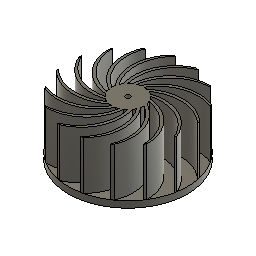
Hélice (Autodesk Fusion 360 design; units mm, degrees)
Autodesk Fusion 360 part; units mm, degrees
sketch "Sketch1" plane through (0, 0, 0) normal (0, 1, 0) x (1, 0, 0)
  circle A0 centre (0, 0) radius 5
  circle A1 centre (0, 0) radius 18.5
  circle A2 centre (0, 0) radius 0.75
  line L0 (-21, 0) -> (20.3872, 0) construction
  line L1 (0, 20) -> (0, -20) construction
  arc A3 (10.124, -15.484) -> (5, 0) centre (-1.6517, -10.791) ccw
  arc A4 (15.2788, -10.4311) -> (4.6194, 1.9134) centre (2.6036, -10.6017) ccw
  arc A5 (18.1076, -3.7901) -> (3.5355, 3.5355) centre (6.4625, -8.7984) ccw
  arc A6 (18.1796, 3.4279) -> (1.9134, 4.6194) centre (9.3375, -5.6555) ccw
  arc A7 (15.484, 10.124) -> (0, 5) centre (10.791, -1.6517) ccw
  arc A8 (10.4311, 15.2788) -> (-1.9134, 4.6194) centre (10.6017, 2.6036) ccw
  arc A9 (3.7901, 18.1076) -> (-3.5355, 3.5355) centre (8.7984, 6.4625) ccw
  arc A10 (-3.4279, 18.1796) -> (-4.6194, 1.9134) centre (5.6555, 9.3375) ccw
  arc A11 (-10.124, 15.484) -> (-5, 0) centre (1.6517, 10.791) ccw
  arc A12 (-15.2788, 10.4311) -> (-4.6194, -1.9134) centre (-2.6036, 10.6017) ccw
  arc A13 (-18.1076, 3.7901) -> (-3.5355, -3.5355) centre (-6.4625, 8.7984) ccw
  arc A14 (-18.1796, -3.4279) -> (-1.9134, -4.6194) centre (-9.3375, 5.6555) ccw
  arc A15 (-15.484, -10.124) -> (0, -5) centre (-10.791, 1.6517) ccw
  arc A16 (-10.4311, -15.2788) -> (1.9134, -4.6194) centre (-10.6017, -2.6036) ccw
  arc A17 (-3.7901, -18.1076) -> (3.5355, -3.5355) centre (-8.7984, -6.4625) ccw
  arc A18 (3.4279, -18.1796) -> (4.6194, -1.9134) centre (-5.6555, -9.3375) ccw
  arc A19 (10.7478, -15.0577) -> (4.9076, 0.9567) centre (-0.8522, -10.2159) ccw
  line L2 (10.7478, -15.0577) -> (10.124, -15.484)
  arc A20 (15.692, -9.7985) -> (4.168, 2.7619) centre (3.1221, -9.7644) ccw
  line L3 (15.692, -9.7985) -> (15.2788, -10.4311)
  arc A21 (18.2472, -3.0476) -> (2.7938, 4.1467) centre (6.6211, -7.8264) ccw
  line L4 (18.2472, -3.0476) -> (18.1076, -3.7901)
  arc A22 (18.0245, 4.1673) -> (0.9942, 4.9002) centre (9.1122, -4.6968) ccw
  line L5 (18.0245, 4.1673) -> (18.1796, 3.4279)
  arc A23 (15.0577, 10.7478) -> (-0.9567, 4.9076) centre (10.2159, -0.8522) ccw
  line L6 (15.0577, 10.7478) -> (15.484, 10.124)
  arc A24 (9.7985, 15.692) -> (-2.7619, 4.168) centre (9.7644, 3.1221) ccw
  line L7 (9.7985, 15.692) -> (10.4311, 15.2788)
  arc A25 (3.0476, 18.2472) -> (-4.1467, 2.7938) centre (7.8264, 6.6211) ccw
  line L8 (3.0476, 18.2472) -> (3.7901, 18.1076)
  arc A26 (-4.1673, 18.0245) -> (-4.9002, 0.9942) centre (4.6968, 9.1122) ccw
  line L9 (-4.1673, 18.0245) -> (-3.4279, 18.1796)
  arc A27 (-10.7478, 15.0577) -> (-4.9076, -0.9567) centre (0.8522, 10.2159) ccw
  line L10 (-10.7478, 15.0577) -> (-10.124, 15.484)
  arc A28 (-15.692, 9.7985) -> (-4.168, -2.7619) centre (-3.1221, 9.7644) ccw
  line L11 (-15.692, 9.7985) -> (-15.2788, 10.4311)
  arc A29 (-18.2472, 3.0476) -> (-2.7938, -4.1467) centre (-6.6211, 7.8264) ccw
  line L12 (-18.2472, 3.0476) -> (-18.1076, 3.7901)
  arc A30 (-18.0245, -4.1673) -> (-0.9942, -4.9002) centre (-9.1122, 4.6968) ccw
  line L13 (-18.0245, -4.1673) -> (-18.1796, -3.4279)
  arc A31 (-15.0577, -10.7478) -> (0.9567, -4.9076) centre (-10.2159, 0.8522) ccw
  line L14 (-15.0577, -10.7478) -> (-15.484, -10.124)
  arc A32 (-9.7985, -15.692) -> (2.7619, -4.168) centre (-9.7644, -3.1221) ccw
  line L15 (-9.7985, -15.692) -> (-10.4311, -15.2788)
  arc A33 (-3.0476, -18.2472) -> (4.1467, -2.7938) centre (-7.8264, -6.6211) ccw
  line L16 (-3.0476, -18.2472) -> (-3.7901, -18.1076)
  arc A34 (4.1673, -18.0245) -> (4.9002, -0.9942) centre (-4.6968, -9.1122) ccw
  line L17 (4.1673, -18.0245) -> (3.4279, -18.1796)
  dimension "d1" = 10
  dimension "d2" = 37
  dimension "d3" = 1.5
  dimension "d5" = 360
  dimension "d7" = 360
  constraint coincident A0.centre A1.centre
  constraint concentric A0 A1
  constraint concentric A1 A2
  constraint horizontal L0
  constraint vertical L1
  constraint coincident A1 A3.start
  constraint coincident A0 A3.end
  constraint coincident L0 A3.end
  constraint coincident A1 A19.start
  constraint coincident A0 A19.end
  measures "d1" diameter of A0
  measures "d2" diameter of A1
  measures "d3" diameter of A2
extrude "Extrude2" add sketch "Sketch1" against normal blind 2 contours A0 | A0 A1 A3 A34 | A0 A3 A19 L2 | A0 A1 A4 A19 | A0 A18 A34 L17 | A1 L2 | A0 A4 A20 L3 | A0 A1 A18 A33 | A1 L17 | A0 A1 A5 A20 | A1 L3 | A0 A17 A33 L16 | A0 A5 A21 L4 | A0 A1 A17 A32 | A1 L16 | A0 A1 A6 A21 | A1 L4 | A0 A16 A32 L15 | A0 A6 A22 L5 | A0 A1 A16 A31 | A1 L15 | A0 A1 A7 A22 | A1 L5 | A0 A15 A31 L14 | A0 A7 A23 L6 | A0 A1 A15 A30 | A1 L14 | A0 A1 A8 A23 | A1 L6 | A0 A14 A30 L13 | A0 A8 A24 L7 | A0 A1 A14 A29 | A1 L13 | A0 A1 A9 A24 | A1 L7 | A0 A13 A29 L12 | A0 A9 A25 L8 | A0 A1 A13 A28 | A1 L12 | A0 A1 A10 A25 | A1 L8 | A0 A12 A28 L11 | A0 A10 A26 L9 | A0 A1 A12 A27 | A1 L11 | A0 A1 A11 A26 | A1 L9 | A0 A11 A27 L10 | A1 L10 | A2 makes body 1
extrude "Extrude1" add sketch "Sketch1" along normal blind 15 separate body contours A0 | A0 A3 A19 L2 | A0 A18 A34 L17 | A0 A4 A20 L3 | A0 A17 A33 L16 | A0 A5 A21 L4 | A0 A16 A32 L15 | A0 A6 A22 L5 | A0 A15 A31 L14 | A0 A7 A23 L6 | A0 A14 A30 L13 | A0 A8 A24 L7 | A0 A13 A29 L12 | A0 A9 A25 L8 | A0 A12 A28 L11 | A0 A10 A26 L9 | A0 A11 A27 L10 makes body 2
extrude "Extrude3" cut sketch "Sketch1" against normal blind 2 contours A2 bodies 1
